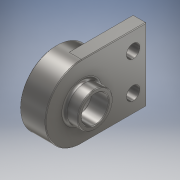
# Autodesk Inventor part: Porta cuscinetto puleggia operatrice
Saved by Autodesk Inventor 2018 (Build 220112000, 112)
## iProperties
Created: 2020-06-12
Part Number: Porta cuscinetto puleggia operatrice
Material: Acciaio inossidabile
Document SubType Name: Modeling
Designer: Francesco
Density: 8 g/cm^3
Appearance: Semilucidato
Author: Francesco
Autodesk Inventor part; units mm, degrees
ref_plane "YZ Plane" through (0, 0, 0) normal (1, 0, 0) x (0, 1, 0)
ref_plane "XZ Plane" through (0, 0, 0) normal (0, 1, 0) x (-1, 0, 0)
ref_plane "XY Plane" through (0, 0, 0) normal (0, 0, 1) x (1, 0, 0)
sketch "Schizzo3" plane through (0, 0, 0) normal (0, 0, 1) x (1, 0, 0)
  line L0 (-66.1458, 0) -> (66.1458, 0)
  line L1 (-4.2292, 27) -> (-4.2292, 13)
  line L2 (-4.2292, 13) -> (5.7708, 13)
  line L3 (5.7708, 13) -> (5.7708, 10)
  line L4 (-23.2292, 27) -> (-23.2292, 23.5)
  line L5 (-23.2292, 23.5) -> (-9.2292, 23.5)
  line L6 (-9.2292, 23.5) -> (-9.2292, 21)
  line L7 (-9.2292, 21) -> (-7.2292, 21)
  line L8 (-7.2292, 21) -> (-7.2292, 10)
  line L9 (-7.2292, 10) -> (5.7708, 10)
  line L10 (-23.2292, 27) -> (-4.2292, 27)
  point P0 (0, 0)
  point P1 (0, 0)
  dimension "d8" = 20
  dimension "d9" = 26
  dimension "d10" = 10
  dimension "d11" = 47
  dimension "d13" = 42
  dimension "d14" = 5
  dimension "d17" = 3
  dimension "d19" = 3.5
  dimension "d21" = 14
  constraints: 22 end point, 7 perpendicular, 2 coincident, 2 horizontal, 1 midpoint, 1 vertical
  measures "d8" diameter of L9 L0
  measures "d9" diameter of L2 L0
  measures "d10" distance between parallel lines of L3 L1
  measures "d11" diameter of L5 L0
  measures "d13" diameter of L7 L0
  measures "d14" distance between parallel lines of L6 L1
  measures "d17" distance between parallel lines of L1 L8
  measures "d19" distance between parallel lines of L5 L10
  measures "d21" distance from line of L6.end L4
revolve "Rivoluzione1" add sketch "Schizzo3" angle 360 about axis through (-66.1458, 0, 0) along (1, 0, 0)
fillet "Raccordo1" radius 2 1 edges at (-4.2292, -13, 0)
chamfer "Smusso1" distance 0.5 angle 45 4 edges at (-23.2292, -23.5, 0) (-7.2292, -10, 0) (5.7708, -10, 0) (5.7708, -13, 0)
sketch "Schizzo4" plane through (-4.2292, 0, 0) normal (1, 0, 0) x (0, 0, -1)
  circle A0 centre (0, 0) radius 27 projected
  circle A1 centre (0, 0) radius 27
  line L0 (-27, 0) -> (-27, 48)
  line L1 (-27, 48) -> (27, 48)
  line L2 (27, 48) -> (27, 0)
  dimension "d27" = 48
  constraints: 6 end point, 3 tangent, 2 perpendicular, 2 point on circle, 1 centre point, 1 coincident, 1 concentric, 1 vertical
  measures "d27" distance of L0.start L0.end
extrude "Estrusione3" add sketch "Schizzo4" against normal blind 9.5 contours A0 L0 L1 L2
chamfer "Smusso2" distance 0.5 angle 45 8 edges at (-4.2292, 24, 27) (-4.2292, -27, 0) (-4.2292, 24, -27) (-23.2292, -27, 0) (-4.2292, 48, 0) (-13.7292, 48, 0) (-8.9792, 48, -27) (-8.9792, 48, 27)
sketch "Schizzo5" plane through (-13.7292, 0, 0) normal (-1, 0, 0) x (0, 0, 1)
  line L0 (27, 0) -> (27, 47.5) projected
  line L1 (26.5, 48) -> (-26.5, 48) projected
  line L2 (-27, 47.5) -> (-27, 0) projected
  point P0 (0, 0)
  point P1 (13.5, 38)
  point P2 (-13.5, 38)
  dimension "d33" = 13.5
  dimension "d34" = 10
  dimension "d35" = 13.5
  constraints: 1 horizontal alignment
  measures "d33" distance from line of L0 point (13.5, 38)
  measures "d34" distance from line of point (13.5, 38) L1
  measures "d35" distance from line of L2 point (-13.5, 38)
hole "Foro1" at (-13.7292, 38, 13.5) at (-13.7292, 38, -13.5) direction (1, 0, 0) diameter 10 end through all
equation "\"d35\" = d33"
